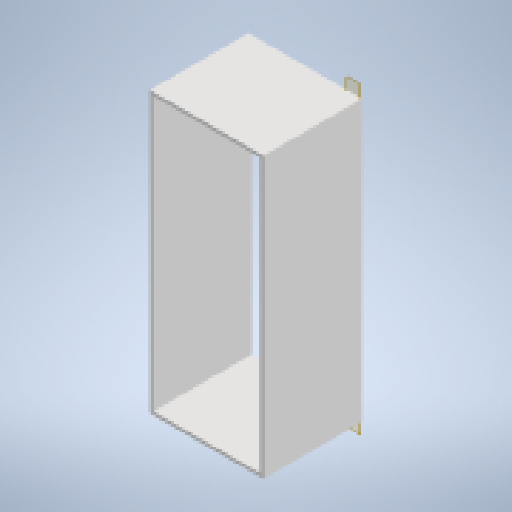
# Autodesk Inventor part: Gear_House
Saved by Autodesk Inventor 2024 (Build 280153000, 153)
## iProperties
Created: 2024-04-16
Part Number: Gear_House
Material: Generic
Document SubType Name: Modeling
Designer: teeta
Density: 1 g/cm^3
Appearance: Default
Author: teeta
Autodesk Inventor part; units mm, degrees
ref_plane "YZ Plane" through (0, 0, 0) normal (1, 0, 0) x (0, 1, 0)
ref_plane "XZ Plane" through (0, 0, 0) normal (0, 1, 0) x (-1, 0, 0)
ref_plane "XY Plane" through (0, 0, 0) normal (0, 0, 1) x (1, 0, 0)
ref_plane "Work Plane1" through (0, 0, 0) normal (0, 0, 1) x (1, 0, 0)
sketch "Sketch1" plane through (0, 0, 0) normal (0, 0, 1) x (1, 0, 0)
  line L0 (-1244.45, -25.4) -> (6.35, -25.4) projected
  line L1 (6.35, 825.4) -> (-1244.45, 825.4) projected
  line L2 (6.35, -25.4) -> (-339.4259, -25.4)
  line L3 (-339.4259, -25.4) -> (-339.4259, 825.4)
  line L4 (-339.4259, 825.4) -> (6.35, 825.4)
  line L5 (6.35, 825.4) -> (6.35, -25.4)
  point P0 (0, 0)
  constraints: 8 end point, 2 parallel, 1 horizontal, 1 perpendicular, 1 point on line
extrude "Extrusion1" add sketch "Sketch1" along normal blind 300
shell "Shell1" thickness 10 removed faces 2 at (-108.9086, 258.2, 0) at (-108.9086, 258.2, 300)
body "Solid1"
